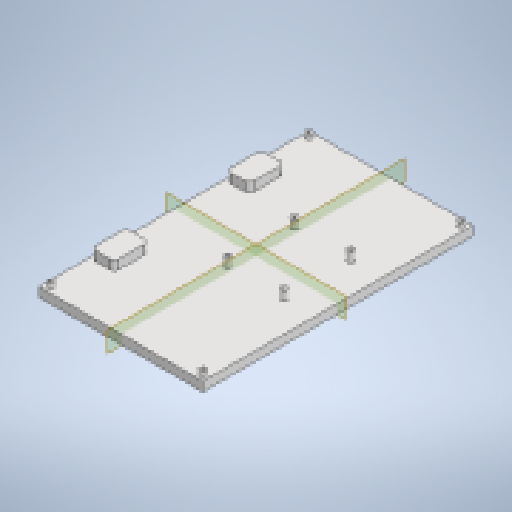
# Autodesk Inventor part: wisecoco-display
Saved by Autodesk Inventor 2024 (Build 280153000, 153)
## iProperties
Created: 2024-08-25
Part Number: wisecoco-display
Material: Generic
Document SubType Name: Modeling
Designer: Stefano
Density: 1 g/cm^3
Appearance: Default
Author: Stefano
Autodesk Inventor part; units mm, degrees
ref_plane "YZ Plane" through (0, 0, 0) normal (1, 0, 0) x (0, 1, 0)
ref_plane "XZ Plane" through (0, 0, 0) normal (0, 1, 0) x (-1, 0, 0)
ref_plane "XY Plane" through (0, 0, 0) normal (0, 0, 1) x (1, 0, 0)
sketch "Sketch1" plane through (0, 0, 0) normal (0, 1, 0) x (-1, 0, 0)
  line L0 (71.25, 117.5) -> (-71.25, 117.5)
  line L1 (-71.25, 117.5) -> (-71.25, -117.5)
  line L2 (-71.25, -117.5) -> (71.25, -117.5)
  line L3 (71.25, -117.5) -> (71.25, 117.5)
  line L4 (71.25, 117.5) -> (-71.25, -117.5) construction
  line L5 (-71.25, 117.5) -> (71.25, -117.5) construction
  point P0 (0, 0)
  dimension "d0" = 235
  dimension "d1" = 142.5
  constraints: 12 end point, 2 midpoint, 2 parallel, 1 horizontal, 1 perpendicular
  measures "d0" distance of L2.end L0.start
  measures "d1" distance of L0.start L0.end
extrude "Extrusion1" add sketch "Sketch1" along normal blind 7.874
sketch "Sketch2" plane through (0, 7.874, 0) normal (0, 1, 0) x (1, 0, 0)
  circle A0 centre (-66.2, -112.45) radius 2.75
  line L0 (-71.25, -117.5) -> (71.25, -117.5) projected
  line L1 (-66.2, -112.45) -> (66.2, -112.45) construction
  line L2 (66.2, -112.45) -> (66.2, 112.45) construction
  line L3 (66.2, 112.45) -> (-66.2, 112.45) construction
  line L4 (-66.2, 112.45) -> (-66.2, -112.45) construction
  line L5 (-66.2, -112.45) -> (66.2, 112.45) construction
  line L6 (66.2, -112.45) -> (-66.2, 112.45) construction
  circle A1 centre (-66.2, 112.45) radius 2.75
  circle A2 centre (66.2, -112.45) radius 2.75
  circle A3 centre (66.2, 112.45) radius 2.75
  line L7 (-71.25, 117.5) -> (-71.25, -117.5) projected
  point P0 (0, 0)
  dimension "d4" = 5.5
  dimension "d6" = 5.5
  dimension "d7" = 5.5
  dimension "d8" = 5.5
  dimension "d45" = 2.3
  dimension "d46" = 2.3
  constraints: 12 end point, 4 centre point, 4 coincident, 2 midpoint, 2 parallel, 1 horizontal, 1 perpendicular
  measures "d4" diameter of A0
  measures "d6" diameter of A1
  measures "d7" diameter of A2
  measures "d8" diameter of A3
  measures "d45" distance edge to line of A0 L7
  measures "d46" distance edge to line of A0 L0
extrude "Extrusion2" add sketch "Sketch2" along normal blind 4
sketch "Sketch3" plane through (-66.2, 11.874, 112.45) normal (0, 1, 0) x (1, 0, 0)
  circle A0 centre (0, 0) radius 2.75 projected
  circle A1 centre (0, 224.9) radius 2.75 projected
  circle A2 centre (132.4, 224.9) radius 2.75 projected
  circle A3 centre (132.4, 0) radius 2.75 projected
  point P0 (66.2, 112.45)
  point P1 (132.4, 0)
  constraints: 4 coincident
hole "Hole1" at (-66.2, 11.874, 112.45) at (-66.2, 11.874, -112.45) at (66.2, 11.874, -112.45) at (66.2, 11.874, 112.45) direction (0, -1, 0) diameter 2.013 depth 4 tip angle 118 thread size "M2.5x0.45" class "6H" standard "ANSI Metric M Profile"
sketch "Sketch4" plane through (0, 7.874, 0) normal (0, 1, 0) x (1, 0, 0)
  line L0 (-69.5, -73.75) -> (-49.5, -73.75)
  line L1 (-49.5, -73.75) -> (-49.5, -43.75)
  line L2 (-49.5, -43.75) -> (-69.5, -43.75)
  line L3 (-69.5, -43.75) -> (-69.5, -73.75)
  line L4 (-69.5, -73.75) -> (-49.5, -43.75) construction
  line L5 (-49.5, -73.75) -> (-69.5, -43.75) construction
  line L6 (-71.25, 117.5) -> (-71.25, -117.5) projected
  line L7 (-71.25, 0) -> (71.25, 0) construction
  line L8 (71.25, -117.5) -> (71.25, 117.5) construction
  line L9 (-69.5, 73.75) -> (-49.5, 73.75)
  line L10 (-49.5, 73.75) -> (-49.5, 43.75)
  line L11 (-49.5, 43.75) -> (-69.5, 43.75)
  line L12 (-69.5, 43.75) -> (-69.5, 73.75)
  line L13 (-69.5, 73.75) -> (-49.5, 43.75) construction
  line L14 (-49.5, 73.75) -> (-69.5, 43.75) construction
  point P0 (0, 0)
  point P1 (-59.5, -58.75)
  point P2 (-59.5, 58.75)
  dimension "d20" = 30
  dimension "d21" = 20
  dimension "d22" = 1.75
  dimension "d23" = 147.5
  constraints: 26 end point, 5 symmetric about line, 4 midpoint, 2 parallel, 1 horizontal, 1 perpendicular
  measures "d20" distance of L2.end L0.start
  measures "d21" distance of L0.start L0.end
  measures "d22" distance between parallel lines of L6 L3
  measures "d23" distance between parallel lines of L9 L0
extrude "Extrusion3" add sketch "Sketch4" along normal blind 8
fillet "Fillet1" radius 4 8 edges at (-49.5, 11.874, 73.75) (-69.5, 11.874, 73.75) (-69.5, 11.874, 43.75) (-49.5, 11.874, 43.75) (-49.5, 11.874, -43.75) (-69.5, 11.874, -43.75) (-69.5, 11.874, -73.75) (-49.5, 11.874, -73.75)
sketch "Sketch5" plane through (0, 7.874, 0) normal (0, 1, 0) x (1, 0, 0)
  line L0 (-4.6, -20.0342) -> (44.4, -20.0342) construction
  line L1 (44.4, -20.0342) -> (44.4, 37.9658) construction
  line L2 (44.4, 37.9658) -> (-4.6, 37.9658) construction
  line L3 (-4.6, 37.9658) -> (-4.6, -20.0342) construction
  line L4 (-4.6, -20.0342) -> (44.4, 37.9658) construction
  line L5 (44.4, -20.0342) -> (-4.6, 37.9658) construction
  circle A0 centre (44.4, 37.9658) radius 2.75
  circle A1 centre (44.4, -20.0342) radius 2.75
  circle A2 centre (-4.6, -20.0342) radius 2.75
  circle A3 centre (-4.6, 37.9658) radius 2.75
  line L6 (71.25, -117.5) -> (71.25, 117.5) projected
  line L7 (71.25, 117.5) -> (-71.25, 117.5) projected
  line L8 (-71.25, -117.5) -> (71.25, -117.5) projected
  point P0 (0, 0)
  point P1 (19.9, 8.9658)
  dimension "d27" = 5.5
  dimension "d28" = 5.5
  dimension "d29" = 63.5
  dimension "d30" = 5.5
  dimension "d31" = 5.5
  dimension "d32" = 24.1
  dimension "d33" = 54.5
  dimension "d34" = 76.7842
  dimension "d44" = 94.7158
  constraints: 12 end point, 4 centre point, 4 coincident, 2 midpoint, 2 parallel, 1 horizontal, 1 perpendicular
  measures "d27" diameter of A0
  measures "d28" diameter of A1
  measures "d30" diameter of A2
  measures "d31" diameter of A3
  measures "d32" distance edge to line of A1 L6
  measures "d34" distance edge to line of A0 L7
  measures "d44" distance edge to line of A2 L8
extrude "Extrusion4" add sketch "Sketch5" along normal blind 8
sketch "Sketch6" plane through (-4.6, 15.874, 20.0342) normal (0, 1, 0) x (1, 0, 0)
  circle A0 centre (0, 58) radius 2.75 projected
  circle A1 centre (49, 58) radius 2.75 projected
  circle A2 centre (49, 0) radius 2.75 projected
  point P0 (4.6, 20.0342)
  point P1 (0, 0)
  point P2 (49, 58)
  constraints: 3 coincident
hole "Hole2" at (-4.6, 15.874, 20.0342) at (-4.6, 15.874, -37.9658) at (44.4, 15.874, -37.9658) at (44.4, 15.874, 20.0342) direction (0, -1, 0) diameter 2.013 depth 8 tip angle 118 thread size "M2.5x0.45" class "6H" standard "ANSI Metric M Profile"
equation "\"d46\" = d45"
body "Solid1"
